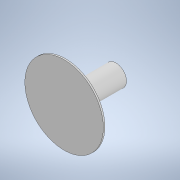
# Autodesk Inventor part: SpringCapV1
Saved by Autodesk Inventor 2020 (Build 240168000, 168)
## iProperties
Created: 2020-06-07
Part Number: SpringCapV1
Material: Generic
Document SubType Name: Modeling
Designer: Kitte_x
Density: 1 g/cm^3
Appearance: Default
Author: Kitte_x
Autodesk Inventor part; units mm, degrees
ref_plane "YZ Plane" through (0, 0, 0) normal (1, 0, 0) x (0, 1, 0)
ref_plane "XZ Plane" through (0, 0, 0) normal (0, 1, 0) x (-1, 0, 0)
ref_plane "XY Plane" through (0, 0, 0) normal (0, 0, 1) x (1, 0, 0)
sketch "Sketch1" plane through (0, 0, 0) normal (0, 0, 1) x (1, 0, 0)
  circle A0 centre (0, 0) radius 1.7
  circle A1 centre (0, 0) radius 2.2
  circle A2 centre (0, 0) radius 3.375
  dimension "d0" = 3.4
  dimension "d1" = 0.5
  dimension "d3" = 6.75
  constraints: 3 centre point, 3 coincident
  measures "d0" diameter of A0
  measures "d1" radial gap between concentric circles of A1 A0
  measures "d3" diameter of A2
extrude "Extrusion1" add sketch "Sketch1" along normal blind 10
sketch "Sketch2" plane through (0, 0, 10) normal (0, 0, 1) x (1, 0, 0)
  circle A0 centre (0, 0) radius 3.375
  dimension "d6" = 6.75
  constraints: 1 centre point, 1 coincident
  measures "d6" diameter of A0
extrude "Extrusion2" add sketch "Sketch2" along normal blind 6
sketch "Sketch3" plane through (0, 0, 16) normal (0, 0, 1) x (1, 0, 0)
  circle A0 centre (0, 0) radius 12.5
  dimension "d12" = 25
  constraints: 1 centre point, 1 coincident
  measures "d12" diameter of A0
extrude "Extrusion3" add sketch "Sketch3" along normal blind 0.5
chamfer "Chamfer2" distance 9.125 distance2 4 1 edges at (-3.375, 0, 16) measured on face at (9.3373, -0.9971, 16)
body "Solid1"
